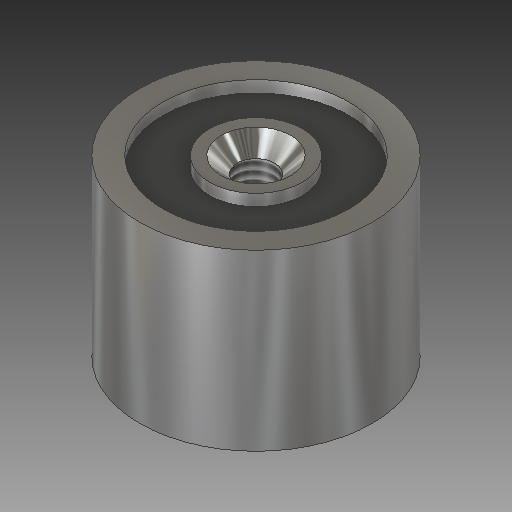
# Autodesk Inventor part: 20-15 Electromagnet
Saved by Autodesk Inventor 2019 (Build 230136000, 136)
## iProperties
Created: 2018-12-14
Part Number: 20-15 Electromagnet
Material: Generic
Document SubType Name: Modeling
Designer: Ax
Density: 1 g/cm^3
Appearance: Chrome - Polished
Mass: 4.42534 g
Surface Area: 17.7671 cm^2
Volume: 4.42534 cm^3
Author: Ax
Autodesk Inventor part; units mm, degrees
ref_plane "YZ Plane" through (0, 0, 0) normal (1, 0, 0) x (0, 1, 0)
ref_plane "XZ Plane" through (0, 0, 0) normal (0, 1, 0) x (-1, 0, 0)
ref_plane "XY Plane" through (0, 0, 0) normal (0, 0, 1) x (1, 0, 0)
sketch "Sketch1" plane through (0, 0, 0) normal (0, 1, 0) x (-1, 0, 0)
  circle A0 centre (0, 0) radius 10
  dimension "d0" = 20
  constraints: 1 centre point, 1 coincident
  measures "d0" diameter of A0
extrude "Extrusion1" add sketch "Sketch1" along normal blind 15
sketch "Sketch2" plane through (0, 15, 0) normal (0, 1, 0) x (1, 0, 0)
  circle A0 centre (0, 0) radius 4
  circle A1 centre (0, 0) radius 8
  circle A2 centre (0, 0) radius 10 projected
  dimension "d3" = 8
  dimension "d4" = 2
  constraints: 2 centre point, 2 coincident
  measures "d3" diameter of A0
  measures "d4" radial gap between concentric circles of A2 A1
extrude "Extrusion2" cut sketch "Sketch2" against normal blind 9 contours A1
sketch "Sketch3" plane through (0, 6, 0) normal (0, 1, 0) x (1, 0, 0)
  circle A0 centre (0, 0) radius 4
  circle A1 centre (0, 0) radius 4 projected
  circle A2 centre (0, 0) radius 8
  circle A3 centre (0, 0) radius 8 projected
  constraints: 3 concentric, 2 centre point, 2 coincident
extrude "Extrusion3" add sketch "Sketch3" along normal blind 8
sketch "Sketch5" plane through (0, 15, 0) normal (0, 1, 0) x (1, 0, 0)
  circle A0 centre (0, 0) radius 4 projected
  circle A1 centre (0, 0) radius 2
  dimension "d20" = 4
  constraints: 1 centre point, 1 coincident
  measures "d20" diameter of A1
hole "Hole2" at (0, 15, 0) direction (0, -1, 0) diameter 3.242 end through all countersink diameter 6 countersink angle 90 thread size "M4x0.7" class "6H" standard "ISO Metric profile"
body "Solid1"
